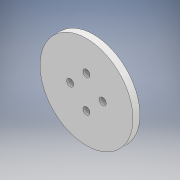
# Autodesk Inventor part: Wrist Sprocket
Saved by Autodesk Inventor 2017 (Build 210142000, 142)
## iProperties
Created: 2018-10-18
Part Number: Wrist Sprocket
Material: Generic
Document SubType Name: Modeling
Designer: Cameron
Density: 1 g/cm^3
Appearance: White
Author: Cameron
Autodesk Inventor part; units mm, degrees
ref_plane "YZ Plane" through (0, 0, 0) normal (1, 0, 0) x (0, 1, 0)
ref_plane "XZ Plane" through (0, 0, 0) normal (0, 1, 0) x (-1, 0, 0)
ref_plane "XY Plane" through (0, 0, 0) normal (0, 0, 1) x (1, 0, 0)
sketch "Sketch1" plane through (0, 0, 0) normal (0, 1, 0) x (-1, 0, 0)
  circle A0 centre (0, 0) radius 20
  line L0 (0, 0) -> (0, 7)
  line L1 (0, 0) -> (-7, 0)
  line L2 (0, 0) -> (0, -7)
  line L3 (0, 0) -> (7, 0)
  circle A1 centre (-7, 0) radius 1.5
  circle A2 centre (0, 7) radius 1.5
  circle A3 centre (0, -7) radius 1.5
  circle A4 centre (7, 0) radius 1.5
  dimension "d0" = 40
  dimension "d1" = 7
  dimension "d2" = 7
  dimension "d3" = 7
  dimension "d4" = 7
  dimension "d5" = 3
  dimension "d6" = 3
  dimension "d8" = 3
  dimension "d11" = 3
  constraints: 8 end point, 5 centre point, 5 coincident, 2 horizontal, 2 vertical
  measures "d0" diameter of A0
  measures "d1" distance of L0.start L0.end
  measures "d2" distance of L0.start L1.end
  measures "d3" distance of L0.start L2.end
  measures "d4" distance of L0.start L3.end
  measures "d5" diameter of A1
  measures "d6" diameter of A2
  measures "d8" diameter of A3
  measures "d11" diameter of A4
extrude "Extrusion2" add sketch "Sketch1" along normal blind 3
body "Solid2"
